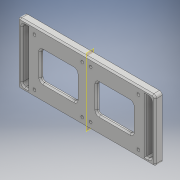
# Autodesk Inventor part: front-stereo2
Saved by Autodesk Inventor 2017 (Build 210142000, 142)
## iProperties
Created: 2017-04-10
Part Number: front-stereo2
Material: Generic
Document SubType Name: Modeling
Designer: Matt Bierner
Density: 1 g/cm^3
Appearance: Default
Author: Matt Bierner
Autodesk Inventor part; units mm, degrees
ref_plane "XZ Plane" through (0, 0, 0) normal (0, 1, 0) x (-1, 0, 0)
ref_plane "XY Plane" through (0, 0, 0) normal (0, 0, 1) x (1, 0, 0)
sketch "Sketch1" plane through (0, 0, 0) normal (0, 1, 0) x (-1, 0, 0)
  line L0 (49, 22) -> (-49, 22)
  line L1 (-49, 22) -> (-49, -22)
  line L2 (-49, -22) -> (49, -22)
  line L3 (49, -22) -> (49, 22)
  line L4 (49, 22) -> (-49, -22) construction
  line L5 (-49, 22) -> (49, -22) construction
  point P0 (0, 0)
  dimension "d0" = 44
  dimension "d1" = 98
  constraints: 12 end point, 2 midpoint, 2 parallel, 1 horizontal, 1 perpendicular
  measures "d0" distance of L2.end L0.start
  measures "d1" distance of L1.end L2.end
extrude "Extrusion1" add sketch "Sketch1" along normal blind 5
sketch "Sketch2" plane through (0, 5, 0) normal (0, 1, 0) x (1, 0, 0)
  line L0 (68.6, 0) -> (-68.6, 0) projected
  line L1 (0, 30.8) -> (0, -30.8) projected
  line L2 (-40, -20) -> (0, -20)
  line L3 (0, -20) -> (0, 20)
  line L4 (0, 20) -> (-40, 20)
  line L5 (-40, 20) -> (-40, -20)
  line L6 (-40, -20) -> (0, 20) construction
  line L7 (0, -20) -> (-40, 20) construction
  point P0 (0, 0)
  point P1 (-20, 0)
  dimension "d4" = 40
  dimension "d5" = 40
  dimension "d6" = 0
  constraints: 12 end point, 2 midpoint, 2 parallel, 1 horizontal, 1 perpendicular, 1 point on line
  measures "d4" distance of L3.end L4.end
  measures "d5" distance of L2.end L3.end
  measures "d6" distance between parallel lines of L1 L3
extrude "Extrusion2" cut sketch "Sketch2" against normal blind 3
sketch "Sketch3" plane through (0, 2, 0) normal (0, 1, 0) x (1, 0, 0)
  line L0 (0, -20) -> (-40, -20) projected
  line L1 (0, 20) -> (0, -20) projected
  line L2 (-40, 20) -> (0, 20) projected
  line L3 (-40, -20) -> (-40, 20) projected
  line L4 (-40, -20) -> (-40, 20) projected
  line L5 (-40, 20) -> (-34, 20)
  line L6 (-34, 20) -> (-34, 14)
  line L7 (-34, 14) -> (-40, 14)
  line L8 (-40, 14) -> (-40, 20)
  line L9 (0, 20) -> (0, -20) projected
  line L10 (0, 20) -> (-6, 20)
  line L11 (-6, 20) -> (-6, 14)
  line L12 (-6, 14) -> (0, 14)
  line L13 (0, 14) -> (0, 20)
  line L14 (0, -20) -> (-40, -20) projected
  line L15 (-40, -20) -> (-34, -20)
  line L16 (-34, -20) -> (-34, -14)
  line L17 (-34, -14) -> (-40, -14)
  line L18 (-40, -14) -> (-40, -20)
  line L19 (0, -20) -> (-6, -20)
  line L20 (-6, -20) -> (-6, -14)
  line L21 (-6, -14) -> (0, -14)
  line L22 (0, -14) -> (0, -20)
  point P0 (0, 0)
  dimension "d9" = 6
  dimension "d10" = 6
  dimension "d11" = 6
  dimension "d12" = 6
  dimension "d13" = 6
  dimension "d14" = 6
  dimension "d15" = 6
  dimension "d38" = 6
  constraints: 32 end point, 8 parallel, 4 horizontal, 4 perpendicular
  measures "d9" distance of L6.end L7.end
  measures "d10" distance of L5.end L6.end
  measures "d11" distance of L12.end L11.end
  measures "d12" distance of L17.end L16.end
  measures "d13" distance of L16.end L15.end
  measures "d14" distance of L20.end L21.end
  measures "d15" distance of L19.end L20.end
  measures "d38" distance of L10.end L11.end
extrude "Extrusion3" add sketch "Sketch3" along normal blind 2 contours L0 L20 L21 L1 | L0 L3 L17 L16 | L12 L11 L2 L1 | L3 L2 L6 L7
sketch "Sketch4" plane through (0, 2, 0) normal (0, 1, 0) x (1, 0, 0)
  line L0 (-40, 20) -> (0, 20) projected
  line L1 (-34, 20) -> (-34, 14) projected
  line L2 (-34, 14) -> (-40, 14) projected
  line L3 (-40, -14) -> (-40, 14) projected
  line L4 (-40, -14) -> (-34, -14) projected
  line L5 (-34, -14) -> (-34, -20) projected
  line L6 (-6, -20) -> (-34, -20) projected
  line L7 (-6, -20) -> (-6, -14) projected
  line L8 (-6, -14) -> (0, -14) projected
  line L9 (0, 14) -> (0, -14) projected
  line L10 (0, 14) -> (-6, 14) projected
  line L11 (-6, 14) -> (-6, 20) projected
  line L12 (-34, 20) -> (-6, 20) projected
  line L13 (-33, -10) -> (-7, -10)
  line L14 (-7, -10) -> (-7, 10)
  line L15 (-7, 10) -> (-33, 10)
  line L16 (-33, 10) -> (-33, -10)
  line L17 (-33, -10) -> (-7, 10) construction
  line L18 (-7, -10) -> (-33, 10) construction
  point P0 (0, 0)
  point P1 (-20, 0)
  dimension "d18" = 26
  dimension "d19" = 20
  dimension "d20" = 20
  dimension "d21" = 20
  constraints: 12 end point, 2 midpoint, 2 parallel, 1 horizontal, 1 perpendicular
  measures "d18" distance of L15.end L14.end
  measures "d19" distance of L14.end L13.end
  measures "d20" distance from line of point (-20, 0) L0
  measures "d21" distance from line of L9 point (-20, 0)
extrude "Extrusion4" cut sketch "Sketch4" against normal through all contours L16 L15 L14 L13
fillet "Fillet1" radius 2 4 edges at (-7, 1, 10) (-7, 1, -10) (-33, 1, 10) (-33, 1, -10)
sketch "Sketch5" plane through (0, 5, 0) normal (0, 1, 0) x (1, 0, 0)
  line L0 (68.6, 0) -> (-68.6, 0) projected
  line L1 (-42, 19) -> (-46, 19)
  line L2 (-46, 19) -> (-46, -19)
  line L3 (-46, -19) -> (-42, -19)
  line L4 (-42, -19) -> (-42, 19)
  line L5 (-42, 19) -> (-46, -19) construction
  line L6 (-46, 19) -> (-42, -19) construction
  line L7 (-40, -20) -> (-40, 20) projected
  point P0 (0, 0)
  point P1 (-44, 0)
  dimension "d25" = 38
  dimension "d26" = 2
  dimension "d27" = 4
  constraints: 12 end point, 2 midpoint, 2 parallel, 1 horizontal, 1 perpendicular, 1 point on line
  measures "d25" distance of L3.end L1.start
  measures "d26" distance between parallel lines of L7 L4
  measures "d27" distance of L2.end L3.end
extrude "Extrusion5" cut sketch "Sketch5" against normal through all
fillet "Fillet2" radius 2 4 edges at (-46, 2.5, 19) (-49, 2.5, 22) (-49, 2.5, -22) (-46, 2.5, -19)
mirror "Mirror1" about plane through (0, 0, 0) normal (1, 0, 0) of "Extrusion2", "Extrusion3", "Extrusion4", "Fillet1", "Extrusion5", "Fillet2"
fillet_without_effect "Fillet3"
chamfer "Chamfer1" distance 1 angle 45 22 edges at (0, 0, 22) (49, 0, 0) (0, 0, -22) (-48.4142, 0, -21.4142) (-49, 0, 0) (-48.4142, 0, 21.4142) (33, 0, 0) (32.4142, 0, -9.4142) (20, 0, -10) (7.5858, 0, -9.4142) (7, 0, 0) (7.5858, 0, 9.4142) (20, 0, 10) (32.4142, 0, 9.4142) (-7, 0, 0) (-7.5858, 0, -9.4142) (-20, 0, -10) (-32.4142, 0, -9.4142) (-33, 0, 0) (-32.4142, 0, 9.4142) (-20, 0, 10) (-7.5858, 0, 9.4142)
chamfer "Chamfer2" distance 1 angle 45 12 edges at (-42, 0, 0) (-45.4142, 0, 18.4142) (-46, 0, 0) (-45.4142, 0, -18.4142) (-43, 0, -19) (-43, 0, 19) (43, 0, 19) (45.4142, 0, 18.4142) (46, 0, 0) (45.4142, 0, -18.4142) (43, 0, -19) (42, 0, 0)
sketch "Sketch6" plane through (0, 0, 0) normal (0, -1, 0) x (1, 0, 0)
  line L0 (-3, 17) -> (-37, 17)
  line L1 (-37, 17) -> (-37, -17)
  line L2 (-37, -17) -> (-3, -17)
  line L3 (-3, -17) -> (-3, 17)
  line L4 (-3, 17) -> (-37, -17) construction
  line L5 (-37, 17) -> (-3, -17) construction
  line L6 (0, 30.8) -> (0, -30.8) projected
  point P0 (0, 0)
  point P1 (-20, 0)
  dimension "d39" = 34
  dimension "d40" = 34
  dimension "d41" = 20
  constraints: 12 end point, 2 midpoint, 2 parallel, 1 horizontal, 1 perpendicular
  measures "d39" distance of L2.end L1.end
  measures "d40" distance of L1.end L0.end
  measures "d41" distance of point (0, 0) point (-20, 0)
hole "Hole1" at (-3, 0, -17) at (-37, 0, -17) at (-37, 0, 17) at (-3, 0, 17) direction (0, 1, 0) diameter 2 depth 8 tip angle 118
mirror "Mirror2" about plane through (0, 0, 0) normal (1, 0, 0) of "Hole1"
body "Solid1"
